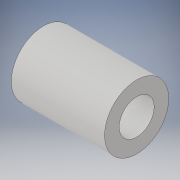
# Autodesk Inventor part: cylinder
Saved by Autodesk Inventor 2017 (Build 210142000, 142)
## iProperties
Created: 2017-01-30
Part Number: cylinder
Material: Generic
Document SubType Name: Modeling
Designer: yul067
Density: 1 g/cm^3
Appearance: Default
Author: yul067
Autodesk Inventor part; units mm, degrees
ref_plane "YZ Plane" through (0, 0, 0) normal (1, 0, 0) x (0, 1, 0)
ref_plane "XZ Plane" through (0, 0, 0) normal (0, 1, 0) x (-1, 0, 0)
ref_plane "XY Plane" through (0, 0, 0) normal (0, 0, 1) x (1, 0, 0)
sketch "Sketch1" plane through (0, 0, 0) normal (1, 0, 0) x (0, 1, 0)
  circle A0 centre (0, 0) radius 11
  dimension "d0" = 22
  constraints: 1 centre point, 1 coincident
  measures "d0" diameter of A0
extrude "Extrusion1" add sketch "Sketch1" along normal blind 32
sketch "Sketch2" plane through (32, 0, 0) normal (1, 0, 0) x (0, 0, -1)
  circle A0 centre (0, 0) radius 6
  dimension "d3" = 12
  constraints: 1 centre point, 1 coincident
  measures "d3" diameter of A0
extrude "Extrusion2" cut sketch "Sketch2" against normal blind 32
body "Solid1"
